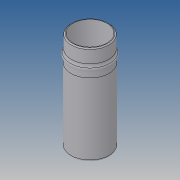
# Autodesk Inventor part: Löffelbox_unten
Saved by Autodesk Inventor 2019.4 (Build 234330000, 330)
## iProperties
Created: 2020-09-25
Part Number: Löffelbox_unten
Material: GEDA Stahl
Document SubType Name: Modeling
Designer: Admin
Mass: 180.343 g
Surface Area: 233.792 cm^2
Volume: 22.9444 cm^3
Density: 7.86 g/cm^3
Appearance: GEDA Stahl A
Gewicht: 0,180 kg
G_L: 0
G_H: 0
G_B: 0
VAULT_Status: In Bearbeitung
Revision: -
Max. Breite: 0
Max. Höhe: 0
Max. Länge: 0
Max. Abmessungen: 0 x 0 x 0
Anfängl. Veröffentlichungsdatum: 2020-02-13
Volumen: 22944,436
InventorVersion: 2019.4
Author: Admin
Autodesk Inventor part; units mm, degrees
note: some values were not read from the file. Left out: dimensions or parameters whose unit could not be read.
ref_plane "YZ Plane" through (0, 0, 0) normal (1, 0, 0) x (0, 1, 0)
ref_plane "XZ Plane" through (0, 0, 0) normal (0, 1, 0) x (-1, 0, 0)
ref_plane "XY Plane" through (0, 0, 0) normal (0, 0, 1) x (1, 0, 0)
sketch "Skizze1" plane through (0, 0, 0) normal (0, 0, 1) x (1, 0, 0)
  circle A0 centre (0, 0) radius 18.75
  circle A1 centre (0, 0) radius 16.75
  dimension "d0" = 37.5
  dimension "d1" = 2
  constraints: 2 centre point, 2 coincident
  measures "d0" diameter of A0
  measures "d1" radial gap between concentric circles of A0 A1
extrude "Extrusion1" add sketch "Skizze1" against normal blind 70
sketch "Skizze2" plane through (0, 0, -70) normal (0, 0, -1) x (-1, 0, 0)
  circle A0 centre (0, 0) radius 18.75 projected
extrude "Extrusion2" add sketch "Skizze2" along normal blind 2
fillet "Rundung1" radius 2 2 edges at (-16.75, 0, -70) (18.75, 0, -72)
sketch "Skizze3" plane through (0, 0, 0) normal (1, 0, 0) x (0, 1, 0)
  line L0 (18.75, 0) -> (18.75, -70) projected
  line L1 (-18.75, 0) -> (18.75, 0) projected
  line L2 (-16.75, 0) -> (16.75, 0) projected
  line L3 (18.75, 0) -> (16.75, 0)
  line L4 (16.75, 0) -> (16.75, 10)
  line L5 (16.75, 10) -> (18.35, 10)
  spline S0 degree 4 poles (18.35, 10) (22.5236, 5.438) (17.0645, 8.0767) (18.75, 3.082) (18.75, 0) knots 0 0 0 0 0 1 1 1 1 1
  line L6 (0, -86.0201) -> (0, 26.1206) projected
  point P0 (0, 0)
  point P1 (19.65, 6.8)
  point P2 (18.75, 5)
  dimension "d7" = 10
  dimension "d8" = 1.6
  dimension "d9" = 2
  dimension "d10" = 2.9
  dimension "d11" = 3.2
  dimension "d12" = 5
  constraints: 6 end point, 2 perpendicular, 1 horizontal, 1 vertical, 4 other
  measures "d7" distance of L2.end L4.end
  measures "d8" distance of L4.end L5.end
  measures "d9" distance from line of L4 point (18.75, 5)
  measures "d10" distance from line of L4 point (19.65, 6.8)
  measures "d11" distance from line of L5 point (19.65, 6.8)
  measures "d12" distance from line of L5 point (18.75, 5)
revolve "Umdrehung1" add sketch "Skizze3" angle 360 about axis through (0, 0, -10) along (0, 0, 1)
sketch "Skizze4" plane through (0, 0, 10) normal (0, 0, 1) x (1, 0, 0)
  circle A0 centre (0, 0) radius 18.35 projected
  circle A1 centre (0, 0) radius 16.75 projected
  point P0 (0, 18.35)
  constraints: 1 vertical alignment
extrude "Extrusion3" add sketch "Skizze4" along normal blind 15
fillet "Rundung2" radius 5 2 edges at (12.9754, 12.9754, 10) (-12.9754, -12.9754, 10)
chamfer "Fase1" distance 1 angle 45 1 edges at (-18.35, 0, 25)
equation "\"G_L\" = 0"
equation "\"G_H\" = 0"
equation "\"G_B\" = 0"
